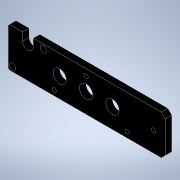
# Autodesk Inventor part: MINI-z-plate-bottom
Saved by Autodesk Inventor 2021 (Build 250183000, 183)
## iProperties
Company: Prusa Development a.s.
Created: 2019-03-18
Material: Všeobecné
Document SubType Name: Modeling
Density: 1 g/cm^3
Appearance: Hliník – tmavý
Project: ORIGINAL PRUSA MINI
Authority: Ing. Robert Turinský
Author: Ing. Robert Turinský
Title: MINI-z-plate-bottom
Revision Number: R4
Autodesk Inventor part; units mm, degrees
ref_plane "YZ Plane" through (0, 0, 0) normal (1, 0, 0) x (0, 1, 0)
ref_plane "XZ Plane" through (0, 0, 0) normal (0, 1, 0) x (-1, 0, 0)
ref_plane "XY Plane" through (0, 0, 0) normal (0, 0, 1) x (1, 0, 0)
sketch "Náčrt1" plane through (0, 0, 0) normal (0, 0, 1) x (1, 0, 0)
  line L0 (0, -21) -> (0, 21) projected
  line L1 (-82.8, 0) -> (83.8, 0) projected
  line L2 (57, -15) -> (-58, -15)
  line L3 (-59, -14) -> (-59, 14)
  line L4 (-58, 15) -> (57, 15)
  line L5 (60, 12) -> (60, -12)
  circle A0 centre (20, 0) radius 5
  circle A1 centre (-20, 0) radius 5
  circle A2 centre (-55.625, -11.625) radius 2.5
  circle A3 centre (-32.375, 11.625) radius 2.5
  circle A4 centre (-24, -11) radius 1.6
  circle A5 centre (0, 10) radius 1.6
  circle A6 centre (51, 0) radius 1.6
  circle A7 centre (31, -11) radius 1.6
  line L6 (6, -6) -> (6, 0)
  line L7 (1, 0) -> (1, -6)
  line L8 (-3.5, -6) -> (-3.5, 0)
  line L9 (-8.5, 0) -> (-8.5, -6)
  arc A8 (1, -6) -> (6, -6) centre (3.5, -6) ccw
  arc A9 (-8.5, -6) -> (-3.5, -6) centre (-6, -6) ccw
  line L10 (-58, -15) -> (-59, -14)
  line L11 (-59, 14) -> (-58, 15)
  line L12 (57, -15) -> (60, -12)
  line L13 (57, 15) -> (60, 12)
  circle A10 centre (0, 0) radius 5
  arc A11 (6, 0) -> (4.4286, 2.3212) centre (3.5, 0) ccw
  arc A12 (1, -4.899) -> (4.4286, 2.3212) centre (0, 0) ccw
  arc A13 (-4.5625, 2.0454) -> (-8.5, 0) centre (-6, 0) ccw
  arc A14 (4.4286, 2.3212) -> (-4.5625, 2.0454) centre (0, 0) ccw
  arc A15 (-3.5, -3.5707) -> (1, -4.899) centre (0, 0) ccw
  arc A16 (-4.5625, 2.0454) -> (-3.5, -3.5707) centre (0, 0) ccw
  arc A17 (1, -4.899) -> (4.4286, 2.3212) centre (0, 0) ccw
  line L14 (1, -4.899) -> (1, -6)
  line L15 (-3.5, -3.5707) -> (-3.5, -6)
  arc A18 (-3.5, 0) -> (-4.5625, 2.0454) centre (-6, 0) ccw
  arc A19 (4.4286, 2.3212) -> (1, 0) centre (3.5, 0) ccw
  line L16 (-48, 15) -> (-48, 9)
  line L17 (-40, 15) -> (-40, 9)
  arc A20 (-48, 9) -> (-40, 9) centre (-44, 9) ccw
  line L18 (-48, 15) -> (-40, 15)
  point P0 (60, -15)
  point P1 (-59, 15)
  point P2 (-59, -15)
  point P3 (60, 15)
  dimension "d0" = 30
  dimension "d1" = 119
  dimension "d2" = 10
  dimension "d3" = 40
  dimension "d5" = 5
  dimension "d6" = 3.375
  dimension "d7" = 3.375
  dimension "d8" = 3.375
  dimension "d9" = 26.625
  dimension "d10" = 40
  dimension "d11" = 35
  dimension "d12" = 4
  dimension "d13" = 3.2
  dimension "d14" = 59
  dimension "d15" = 5
  dimension "d16" = 9
  dimension "d17" = 29
  dimension "d18" = 5
  dimension "d19" = 4.5
  dimension "d21" = 50.5
  dimension "d22" = 6.5
  dimension "d23" = 1
  dimension "d24" = 1
  dimension "d25" = 1
  dimension "d26" = 1
  dimension "d27" = 3
  dimension "d28" = 3
  dimension "d29" = 3
  dimension "d30" = 3
  dimension "d33" = 10
  dimension "d34" = 8
  dimension "d35" = 10
  dimension "d36" = 15
  constraints: 34 end point, 28 point on circle, 21 centre point, 15 point on line, 13 equal radius, 13 tangent, 6 parallel, 4 horizontal alignment, 4 vertical, 2 horizontal, 2 vertical alignment, 1 coincident, 1 collinear, 1 perpendicular, 1 symmetric about line, 2 other
  measures "d0" distance between parallel lines of L4 L2
  measures "d1" distance between parallel lines of L3 L5
  measures "d2" diameter of A0
  measures "d3" distance of A1.centre A0.centre
  measures "d5" diameter of A2
  measures "d6" distance from line of L2 A2.centre
  measures "d7" distance from line of L3 A2.centre
  measures "d8" distance from line of L4 A3.centre
  measures "d9" distance from line of L3 A3.centre
  measures "d10" distance from line of A0.centre L5
  measures "d11" distance from line of L3 A4.centre
  measures "d12" distance from line of L2 A4.centre
  measures "d13" diameter of A4
  measures "d14" distance from line of L3 A5.centre
  measures "d15" distance from line of L4 A5.centre
  measures "d16" distance from line of L5 A6.centre
  measures "d17" distance from line of A7.centre L5
  measures "d18" distance between parallel lines of L7 L6
  measures "d19" distance between parallel lines of L7 L8
  measures "d21" distance between parallel lines of L9 L3
  measures "d22" distance edge to line of A9 L2
  measures "d23" distance of L2.end point (-59, -15)
  measures "d24" distance of L3.start point (-59, -15)
  measures "d25" distance of L3.end point (-59, 15)
  measures "d26" distance of L4.start point (-59, 15)
  measures "d27" distance of L2.start point (60, -15)
  measures "d28" distance of L5.end point (60, -15)
  measures "d29" distance of L4.end point (60, 15)
  measures "d30" distance of L5.start point (60, 15)
  measures "d33" diameter of A10
  measures "d34" distance between parallel lines of L16 L17
  measures "d36" distance from line of L3 A20.centre
extrude "Vysunutí1" add sketch "Náčrt1" along normal blind 5 contours L2 L10 L3 L1 A1 L9 A9 L8 A10 L0 | L0 A10 L7 A8 L6 L1 A0 A6 L5 L12 L2 | L8 A9 L9 L1 A10 | A10 L1 L6 A8 L7 | A10 A13 L1 A1 L3 L11 L4 L16 A20 L17 L0 A5 | L0 A5 L4 L13 L5 L1 A6 A0 A11 A10 | L1 A13 A10 | A10 A11 L1
equation "\"d7\" = d6"
equation "\"d8\" = d6"
equation "\"d24\" = d23"
equation "\"d25\" = d23"
equation "\"d26\" = d25"
equation "\"d28\" = d27"
equation "\"d29\" = d27"
equation "\"d30\" = d29"
